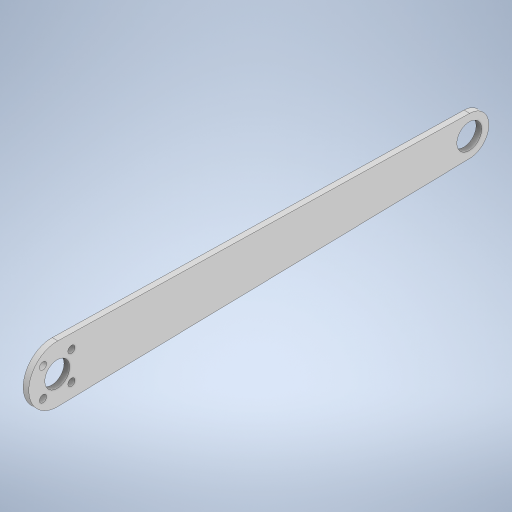
# Autodesk Inventor part: arm
Saved by Autodesk Inventor 2023 (Build 270158000, 158)
## iProperties
Created: 2022-09-10
Part Number: arm
Material: Generic
Document SubType Name: Modeling
Designer: deli
Density: 1 g/cm^3
Appearance: Default
Mass: 20.635 g
Surface Area: 151.802 cm^2
Volume: 20.635 cm^3
Author: deli
Autodesk Inventor part; units mm, degrees
ref_plane "YZ Plane" through (0, 0, 0) normal (1, 0, 0) x (0, 1, 0)
ref_plane "XZ Plane" through (0, 0, 0) normal (0, 1, 0) x (-1, 0, 0)
ref_plane "XY Plane" through (0, 0, 0) normal (0, 0, 1) x (1, 0, 0)
sketch "Sketch1" plane through (0, 0, 0) normal (1, 0, 0) x (0, 1, 0)
  circle A0 centre (62.0682, -4.1091) radius 2
  circle A1 centre (62.0682, -20.1091) radius 2
  circle A2 centre (46.0682, -20.1091) radius 2
  circle A3 centre (46.0682, -4.1091) radius 2
  line L0 (62.0682, -4.1091) -> (62.0682, -20.1091) construction
  line L1 (62.0682, -20.1091) -> (46.0682, -20.1091) construction
  line L2 (46.0682, -20.1091) -> (46.0682, -4.1091) construction
  line L3 (46.0682, -4.1091) -> (62.0682, -4.1091) construction
  circle A4 centre (54.0682, -12.1091) radius 7
  line L4 (62.0682, -4.1091) -> (46.0682, -20.1091) construction
  line L5 (62.0682, -20.1091) -> (46.0682, -4.1091) construction
  arc A5 (70.0644, -12.4539) -> (38.0719, -12.4539) centre (54.0682, -12.1091) ccw
  circle A6 centre (54.0682, -244.1091) radius 7
  line L6 (54.0682, -12.1091) -> (54.0682, -244.1091) construction
  arc A7 (43.0707, -244.3462) -> (65.0656, -244.3462) centre (54.0682, -244.1091) ccw
  line L7 (70.0644, -12.4539) -> (65.0656, -244.3462)
  line L8 (43.0707, -244.3462) -> (38.0719, -12.4539)
  line L9 (40.0714, -12.4108) -> (45.0702, -244.3031)
  arc A8 (42.1281, -4.7992) -> (40.0714, -12.4108) centre (54.0682, -12.1091) ccw
  arc A9 (68.0649, -12.4108) -> (66.0082, -4.7992) centre (54.0682, -12.1091) ccw
  arc A10 (61.3781, -0.1691) -> (46.7582, -0.1691) centre (54.0682, -12.1091) ccw
  line L10 (58.1952, -3.1091) -> (49.9411, -3.1091)
  arc A11 (61.3781, -0.1691) -> (58.1952, -3.1091) centre (62.0682, -4.1091) ccw
  arc A12 (63.0682, -7.9821) -> (66.0082, -4.7992) centre (62.0682, -4.1091) ccw
  arc A13 (42.1281, -4.7992) -> (45.0682, -7.9821) centre (46.0682, -4.1091) ccw
  arc A14 (49.9411, -3.1091) -> (46.7582, -0.1691) centre (46.0682, -4.1091) ccw
  line L11 (45.0682, -7.9821) -> (45.0682, -16.2361)
  line L12 (63.0682, -7.9821) -> (63.0682, -16.2361)
  line L13 (46.0682, -20.1091) -> (40.309, -23.4341) construction
  line L14 (40.309, -23.4341) -> (67.489, -39.1265) construction
  line L15 (67.489, -39.1265) -> (40.9773, -54.4331) construction
  line L16 (40.9773, -54.4331) -> (66.8372, -69.3633) construction
  line L17 (66.8372, -69.3633) -> (41.613, -83.9265) construction
  line L18 (41.613, -83.9265) -> (66.217, -98.1316) construction
  line L19 (42.218, -111.9875) -> (66.217, -98.1316) construction
  line L20 (42.218, -111.9875) -> (65.627, -125.5027) construction
  line L21 (65.627, -125.5027) -> (42.7935, -138.6856) construction
  line L22 (42.7935, -138.6856) -> (65.0656, -151.5445) construction
  line L23 (65.0656, -151.5445) -> (43.3411, -164.0872) construction
  line L24 (43.3411, -164.0872) -> (64.5315, -176.3215) construction
  line L25 (64.5315, -176.3215) -> (43.862, -188.255) construction
  line L26 (43.862, -188.255) -> (64.0234, -199.8952) construction
  line L27 (64.0234, -199.8952) -> (44.3577, -211.2491) construction
  line L28 (44.3577, -211.2491) -> (63.5399, -222.324) construction
  line L29 (63.5399, -222.324) -> (44.8293, -233.1265) construction
  line L30 (44.8293, -233.1265) -> (49.9794, -236.0999) construction
  line L31 (48.9928, -236.6767) -> (44.8543, -234.2874)
  line L32 (44.8045, -231.9777) -> (61.5398, -222.3155)
  line L33 (61.5398, -222.3155) -> (44.3827, -212.4099)
  line L34 (44.3329, -210.1001) -> (62.0231, -199.8868)
  line L35 (62.0231, -199.8868) -> (43.8871, -189.4159)
  line L36 (43.8373, -187.1062) -> (62.531, -176.3134)
  line L37 (62.531, -176.3134) -> (43.3661, -165.2485)
  line L38 (43.3163, -162.9387) -> (63.0648, -151.5369)
  line L39 (63.0648, -151.5369) -> (42.8185, -139.8477)
  line L40 (42.7687, -137.538) -> (63.6259, -125.4961)
  line L41 (63.6259, -125.4961) -> (42.243, -113.1507)
  line L42 (42.1932, -110.841) -> (64.2156, -98.1263)
  line L43 (64.2156, -98.1263) -> (41.6382, -85.0913)
  line L44 (41.5884, -82.7815) -> (64.8354, -69.3598)
  line L45 (64.8354, -69.3598) -> (41.0024, -55.5998)
  line L46 (40.9526, -53.2901) -> (65.4868, -39.1253)
  line L47 (65.4868, -39.1253) -> (40.3342, -24.6034)
  line L48 (40.2844, -22.2936) -> (42.2141, -21.1796)
  line L49 (51.1311, -235.6018) -> (46.8292, -233.1181)
  line L50 (46.8292, -233.1181) -> (63.5148, -223.4848)
  line L51 (63.5646, -221.1749) -> (46.3579, -211.2406)
  line L52 (46.3579, -211.2406) -> (63.9983, -201.056)
  line L53 (64.0481, -198.7461) -> (45.8625, -188.2466)
  line L54 (45.8625, -188.2466) -> (64.5065, -177.4826)
  line L55 (64.5563, -175.1726) -> (45.3418, -164.0792)
  line L56 (45.3418, -164.0792) -> (65.0406, -152.7062)
  line L57 (65.0904, -150.3962) -> (44.7945, -138.6784)
  line L58 (44.7945, -138.6784) -> (65.6019, -126.6654)
  line L59 (65.6517, -124.3554) -> (44.2193, -111.9814)
  line L60 (44.2193, -111.9814) -> (66.192, -99.2956)
  line L61 (66.2417, -96.9856) -> (43.6148, -83.9219)
  line L62 (43.6148, -83.9219) -> (66.8121, -70.5291)
  line L63 (66.8619, -68.2191) -> (42.9793, -54.4305)
  line L64 (42.9793, -54.4305) -> (67.4638, -40.2945)
  line L65 (67.5136, -37.986) -> (42.309, -23.4341)
  arc A15 (45.0682, -16.2361) -> (42.2141, -21.1796) centre (46.0682, -20.1091) ccw
  arc A16 (43.2016, -22.9239) -> (49.9592, -21.1091) centre (46.0682, -20.1091) ccw
  line L66 (42.309, -23.4341) -> (43.2016, -22.9239)
  arc A17 (63.0661, -244.303) -> (51.1311, -235.6018) centre (54.0682, -244.1091) ccw
  arc A18 (48.9928, -236.6767) -> (45.0702, -244.3031) centre (54.0682, -244.1091) ccw
  arc A19 (67.7967, -24.8527) -> (64.5542, -23.2428) centre (65.7972, -24.8096) ccw
  arc A20 (64.6869, -17.0855) -> (67.9958, -15.6168) centre (65.9963, -15.5737) ccw
  line L67 (63.0661, -244.303) -> (67.7967, -24.8527)
  line L68 (67.9958, -15.6168) -> (68.0649, -12.4108)
  arc A21 (58.1952, -21.1091) -> (64.5542, -23.2428) centre (62.0682, -20.1091) ccw
  arc A22 (64.6869, -17.0855) -> (63.0682, -16.2361) centre (62.0682, -20.1091) ccw
  line L69 (58.1952, -21.1091) -> (49.9592, -21.1091)
  circle A23 centre (42.1401, -15.5737) radius 2
  point P0 (0, 0)
  dimension "d0" = 4
  dimension "d1" = 4
  dimension "d2" = 4
  dimension "d3" = 4
  dimension "d4" = 16
  dimension "d5" = 16
  dimension "d6" = 14
  dimension "d7" = 32
  dimension "d8" = 14
  dimension "d9" = 232
  dimension "d10" = 4
  dimension "d18" = 2
  dimension "d19" = 2
  dimension "d20" = 1
  dimension "d21" = 2
  dimension "d22" = 2
  dimension "d23" = 1
  dimension "d24" = 1
  dimension "d25" = 2
  dimension "d26" = 2
  dimension "d27" = 2
  dimension "d29" = 120
  dimension "d30" = 60
  dimension "d31" = 60
  dimension "d33" = 1
  dimension "d34" = 1
  dimension "d35" = 4
  dimension "d36" = 4
  dimension "d37" = 1
  dimension "d38" = 4
  dimension "d39" = 2
  constraints: 136 end point, 46 parallel, 34 point on circle, 24 centre point, 7 tangent, 4 vertical, 3 coincident, 3 perpendicular, 1 horizontal, 1 midpoint, 61 other
  measures "d0" diameter of A0
  measures "d1" diameter of A3
  measures "d2" diameter of A2
  measures "d3" diameter of A1
  measures "d4" distance of L0.start L0.end
  measures "d5" distance of L2.end L0.start
  measures "d6" diameter of A4
  measures "d7" diameter of A5
  measures "d8" diameter of A6
  measures "d9" distance of L6.start L6.end
  measures "d10" radial gap between concentric circles of A7 A6
  measures "d18" radial gap between concentric circles of A5 A10
  measures "d19" radial gap between concentric circles of A5 A9
  measures "d20" distance between parallel lines of L3 L10
  measures "d21" radial gap between concentric circles of A3 A14
  measures "d22" radial gap between concentric circles of A0 A11
  measures "d23" distance between parallel lines of L2 L11
  measures "d24" distance between parallel lines of L0 L12
  measures "d25" radial gap between concentric circles of A12 A0
  measures "d26" radial gap between concentric circles of A13 A3
  measures "d27" radial gap between concentric circles of A5 A8
  measures "d29" angle of L2 L13
  measures "d30" angle of L14 L13
  measures "d31" angle of L15 L14
  measures "d33" distance between parallel lines of L14 L47
  measures "d34" distance between parallel lines of L14 L65
  measures "d35" diameter of A19
  measures "d36" diameter of A20
  measures "d37" distance between parallel lines of L69 L1
  measures "d38" diameter of A23
  measures "d39" radial gap between concentric circles of A2 A15
extrude "Extrusion1" add sketch "Sketch1" along normal blind 3.175 contours L7 A7 L8 A5 | L47 L46 L9 | L45 L44 L9 | L43 L42 L9 | L41 L40 L9 | L39 L38 L9 | L37 L36 L9 | L35 L34 L9 | L33 L32 L9 | L31 A18 L9 | A8 A13 L11 A15 A23 L9 | A23 A15 L48 L9 | A23 | L68 A20 A22 L12 A12 A9 | A11 L10 A14 A10 | L49 L50 L67 A17 | L51 L52 L67 | L53 L54 L67 | L55 L56 L67 | L57 L58 L67 | L59 L60 L67 | L61 L62 L67 | L63 L64 L67 | L65 L66 A16 L69 A21 A19 L67
equation "\"d1\" = d0"
equation "\"d2\" = d0"
equation "\"d3\" = d0"
equation "\"d31\" = d30"
body "Solid1"
